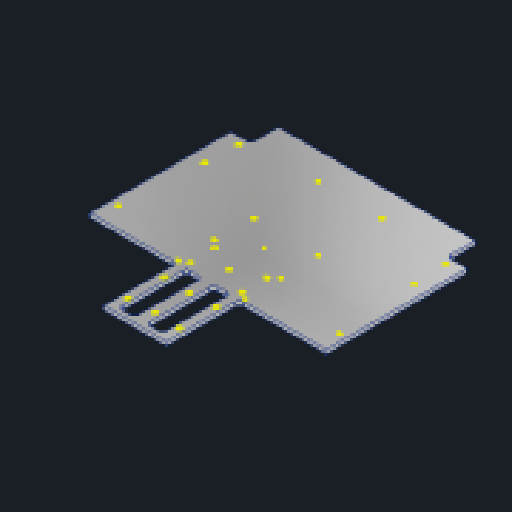
# Autodesk Inventor part: base
Saved by Autodesk Inventor 2023 (Build 270158000, 158)
## iProperties
Created: 2024-04-10
Part Number: base
Material: Aluminum 6061
Document SubType Name: Modeling
Designer: szymo
Density: 2.7 g/cm^3
Appearance: Aluminum - Flat
Mass: 138.037 g
Surface Area: 408.524 cm^2
Volume: 51.1249 cm^3
Author: szymo
Autodesk Inventor part; units mm, degrees
ref_plane "YZ Plane" through (0, 0, 0) normal (1, 0, 0) x (0, 1, 0)
ref_plane "XZ Plane" through (0, 0, 0) normal (0, 1, 0) x (-1, 0, 0)
ref_plane "XY Plane" through (0, 0, 0) normal (0, 0, 1) x (1, 0, 0)
sketch "Sketch2" plane through (0, 0, 0) normal (0, 1, 0) x (-1, 0, 0)
  line L0 (-89, 99) -> (89, 99)
  line L1 (89, 99) -> (89, -99)
  line L2 (89, -99) -> (-89, -99)
  line L3 (-89, -99) -> (-89, 99)
  line L4 (-89, 99) -> (89, -99) construction
  line L5 (89, 99) -> (-89, -99) construction
  line L6 (-89, 99) -> (89, 99)
  line L7 (89, 99) -> (89, -85)
  line L8 (89, -85) -> (-89, -85)
  line L9 (-89, -85) -> (-89, 99)
  line L10 (-4.5, 99) -> (-89, 99)
  line L11 (-89, 99) -> (-89, 42)
  line L12 (-89, 42) -> (-4.5, 42)
  line L13 (-4.5, 42) -> (-4.5, 99)
  line L14 (4.5, 99) -> (89, 99)
  line L15 (89, 99) -> (89, 42)
  line L16 (89, 42) -> (4.5, 42)
  line L17 (4.5, 42) -> (4.5, 99)
  line L18 (22.5, 77.5) -> (22.5, 66.5) projected
  line L19 (16.5, 66.5) -> (16.5, 77.5) projected
  line L20 (-22.5, 66.5) -> (-22.5, 77.5) projected
  line L21 (-16.5, 77.5) -> (-16.5, 66.5) projected
  line L22 (-23.5, 99) -> (-16.5, 99)
  line L23 (-16.5, 99) -> (-16.5, 42)
  line L24 (-16.5, 42) -> (-23.5, 42)
  line L25 (-23.5, 42) -> (-23.5, 99)
  line L26 (16.5, 99) -> (23.5, 99)
  line L27 (23.5, 99) -> (23.5, 42)
  line L28 (23.5, 42) -> (16.5, 42)
  line L29 (16.5, 42) -> (16.5, 99)
  line L30 (-89, 99) -> (89, 99)
  line L31 (89, 99) -> (89, 97)
  line L32 (89, 97) -> (-89, 97)
  line L33 (-89, 97) -> (-89, 99)
  line L34 (89, -85) -> (74, -85)
  line L35 (74, -85) -> (74, -64)
  line L36 (74, -64) -> (89, -64)
  line L37 (89, -64) -> (89, -85)
  line L38 (-89, -85) -> (-74, -85)
  line L39 (-74, -85) -> (-74, -64)
  line L40 (-74, -64) -> (-89, -64)
  line L41 (-89, -64) -> (-89, -85)
  line L42 (16.5, 97) -> (-16.5, 97)
  line L43 (-16.5, 97) -> (-16.5, 93)
  line L44 (-16.5, 93) -> (16.5, 93)
  line L45 (16.5, 93) -> (16.5, 97)
  line L46 (-84.4, -75) -> (-84.4, -71.5) projected
  line L47 (-84.4, -71.5) -> (-87, -71.5) projected
  line L48 (-87, -71.5) -> (-87, -75) projected
  line L49 (-87, -75) -> (-84.4, -75) projected
  line L50 (-79.6, -75) -> (-77, -75) projected
  line L51 (-77, -75) -> (-77, -71.5) projected
  line L52 (-77, -71.5) -> (-79.6, -71.5) projected
  line L53 (-79.6, -71.5) -> (-79.6, -75) projected
  line L54 (-75, -78) -> (-89, -78) projected
  line L55 (-89, -78) -> (-89, -63) projected
  line L56 (-89, -63) -> (-75, -63) projected
  line L57 (-75, -63) -> (-75, -78) projected
  circle A0 centre (-80.45, -67.25) radius 1.25 projected
  point P0 (0, 0)
  point P1 (4.5, 99)
  point P2 (-4.5, 99)
  point P3 (-89, 42)
  point P4 (89, 42)
  point P5 (4.5, 97)
  point P6 (-4.5, 97)
  point P7 (-16.5, 97)
  point P8 (-23.5, 97)
  point P9 (23.5, 97)
  point P10 (16.5, 98)
  point P11 (-4.5, 93)
  point P12 (4.5, 93)
  point P13 (16.5, 93)
  dimension "d8" = 178
  dimension "d9" = 198
  dimension "d10" = 14
  dimension "d11" = 84.5
  dimension "d13" = 84.5
  dimension "d17" = 9
  dimension "d18" = 2
  dimension "d19" = 15
  dimension "d20" = 21
  dimension "d21" = 15
  dimension "d22" = 21
  dimension "d75" = 55
  dimension "d76" = 55
  dimension "d77" = 7
  dimension "d78" = 7
  dimension "d79" = 4
  constraints: 84 end point, 20 parallel, 10 horizontal, 10 perpendicular, 10 point on line, 2 collinear, 2 midpoint, 5 other
  measures "d8" distance of L1.end L2.end
  measures "d9" distance of L0.end L1.end
  measures "d10" distance between parallel lines of L8 L2
  measures "d11" distance of L12.end L11.end
  measures "d13" distance of L15.end L16.end
  measures "d17" distance between parallel lines of L13 L17
  measures "d18" distance of L30.end L31.end
  measures "d19" distance of L35.end L36.end
  measures "d20" distance of L34.end L35.end
  measures "d21" distance of L40.end L39.end
  measures "d22" distance of L39.end L38.end
  measures "d75" distance between parallel lines of L32 L12
  measures "d76" distance between parallel lines of L32 L16
  measures "d77" distance between parallel lines of L23 L25
  measures "d78" distance between parallel lines of L27 L29
  measures "d79" distance of L43.end L42.end
extrude "Extrusion2" add sketch "Sketch2" along normal blind 3 contours L32 L23 L21 L12 L25 | L12 L13 L44 L17 L16 L1 L36 L35 L8 L39 L40 L57 L56 L3 | L32 L13 L44 L23 | L56 L57 L40 L3 | L32 L17 L44 L13 | L32 L29 L44 L17 | L32 L27 L16 L29 L19
fillet "Fillet5" radius 3 12 edges at (-16.5, 1.5, 42) (-4.5, 1.5, 42) (-23.5, 1.5, 42) (16.5, 1.5, 42) (-16.5, 1.5, 93) (-4.5, 1.5, 93) (4.5, 1.5, 93) (16.5, 1.5, 93) (4.5, 1.5, 42) (23.5, 1.5, 42) (74, 1.5, -64) (-74, 1.5, -64)
sketch "Sketch6" plane through (0, 3, 0) normal (0, 1, 0) x (1, 0, 0)
  circle A0 centre (79, 33.8889) radius 1.8 projected
  circle A1 centre (78, 58.6725) radius 1.8 projected
  circle A2 centre (-78, 58.6725) radius 1.8 projected
  circle A3 centre (-79, 33.8889) radius 1.8 projected
  circle A4 centre (-25, -39.7) radius 1.5 projected
  circle A5 centre (-25, -12.55) radius 1.5 projected
  circle A6 centre (-83.35, -26.625) radius 1.5 projected
  circle A7 centre (25, -12.55) radius 1.5 projected
  circle A8 centre (25, -39.7) radius 1.5 projected
  circle A9 centre (83.35, -26.625) radius 1.5 projected
  circle A10 centre (19.5, -17.75) radius 1.8 projected
  circle A11 centre (19.5, -36.375) radius 1.8 projected
  circle A12 centre (19.5, -55.8) radius 1.8 projected
  circle A13 centre (19.4231, -83.3077) radius 1.8 projected
  circle A14 centre (0, -82.2) radius 1.8 projected
  circle A15 centre (-19.4231, -83.3077) radius 1.8 projected
  circle A16 centre (-19.5, -55.8) radius 1.8 projected
  circle A17 centre (0, -56.55) radius 1.8 projected
  circle A18 centre (0, -26.625) radius 1.8 projected
  circle A19 centre (-19.5, -17.75) radius 1.8 projected
  circle A20 centre (-19.5, -36.375) radius 1.8 projected
  circle A21 centre (24.1, 16.4) radius 1.6 projected
  circle A22 centre (24.1, 64.6) radius 1.6 projected
  circle A23 centre (-24.1, 64.6) radius 1.6 projected
  circle A24 centre (-24.1, 16.4) radius 1.6 projected
  point P0 (0, 0)
equation "\"d11\" = d13"
body "Solid2"
